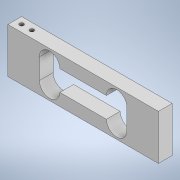
# Autodesk Inventor part: load_cell
Saved by Autodesk Inventor 2022 (Build 260153000, 153)
## iProperties
Created: 2022-01-31
Part Number: load_cell
Material: Generic
Document SubType Name: Modeling
Designer: Martijn
Density: 1 g/cm^3
Appearance: Default
Author: Martijn
Autodesk Inventor part; units mm, degrees
ref_plane "YZ Plane" through (0, 0, 0) normal (1, 0, 0) x (0, 1, 0)
ref_plane "XZ Plane" through (0, 0, 0) normal (0, 1, 0) x (-1, 0, 0)
ref_plane "XY Plane" through (0, 0, 0) normal (0, 0, 1) x (1, 0, 0)
sketch "Sketch1" plane through (0, 0, 0) normal (0, 0, 1) x (1, 0, 0)
  line L0 (0, 0) -> (110, 0)
  line L1 (110, 0) -> (110, 33)
  line L2 (110, 33) -> (0, 33)
  line L3 (0, 33) -> (0, 0)
  dimension "d0" = 33
  dimension "d1" = 110
  constraints: 8 end point, 2 parallel, 1 horizontal, 1 perpendicular
  measures "d0" distance of L2.end L0.start
  measures "d1" distance of L1.end L2.end
extrude "Extrusion1" add sketch "Sketch1" along normal blind 10
sketch "Sketch2" plane through (0, 0, 10) normal (0, 0, 1) x (1, 0, 0)
  arc A0 (38, 24) -> (23, 24) centre (30.5, 24) ccw
  line L0 (23, 24) -> (23, 9)
  arc A1 (23, 9) -> (38, 9) centre (30.5, 9) ccw
  line L1 (38, 24) -> (55, 24)
  line L2 (55, 24) -> (55, 9)
  line L3 (55, 9) -> (38, 9)
  line L4 (0, 0) -> (110, 0) projected
  line L5 (55, 0) -> (55, 9)
  dimension "d4" = 7.5
  dimension "d5" = 15
  dimension "d6" = 9
  dimension "d7" = 17
  dimension "d8" = 7.5
  constraints: 10 end point, 4 point on circle, 4 point on line, 2 centre point, 2 perpendicular, 1 collinear, 1 horizontal, 1 midpoint, 1 vertical
  measures "d4" radius of A0
  measures "d5" distance between parallel lines of L3 L1
  measures "d6" distance between parallel lines of L4 L3
  measures "d7" distance from line of L1.start L2
  measures "d8" radius of A1
extrude "Extrusion2" cut sketch "Sketch2" against normal blind 10
sketch "Sketch3" plane through (0, 33, 0) normal (0, 1, 0) x (1, 0, 0)
  circle A0 centre (5, -5) radius 1.5
  circle A1 centre (12.5, -5) radius 1.5
  line L0 (0, 0) -> (0, -10) projected
  line L1 (110, -10) -> (0, -10) projected
  dimension "d11" = 3
  dimension "d12" = 3
  dimension "d13" = 7.5
  dimension "d14" = 5
  dimension "d15" = 5
  dimension "d16" = 5
  constraints: 2 centre point
  measures "d11" diameter of A0
  measures "d12" diameter of A1
  measures "d13" distance of A1.centre A0.centre
  measures "d14" distance from line of L0 A0.centre
  measures "d15" distance from line of L1 A0.centre
  measures "d16" distance from line of L1 A1.centre
extrude "Extrusion3" cut sketch "Sketch3" against normal blind 13
mirror "Mirror1" about plane through (55, 24, 10) normal (-1, 0, 0) of "Extrusion2"
sketch "Sketch4" plane through (0, 0, 0) normal (0, -1, 0) x (1, 0, 0)
  circle A0 centre (105, 5) radius 1.5
  circle A1 centre (97.5, 5) radius 1.5
  line L0 (110, 0) -> (110, 10) projected
  line L1 (0, 0) -> (110, 0) projected
  dimension "d19" = 3
  dimension "d20" = 5
  dimension "d21" = 5
  dimension "d22" = 7.5
  dimension "d23" = 5
  constraints: 2 centre point, 1 equal radius
  measures "d19" diameter of A1
  measures "d20" distance from line of L0 A0.centre
  measures "d21" distance from line of L1 A0.centre
  measures "d22" distance of A1.centre A0.centre
  measures "d23" distance from line of L1 A1.centre
extrude "Extrusion4" cut sketch "Sketch4" against normal blind 13
body "Solid1"
